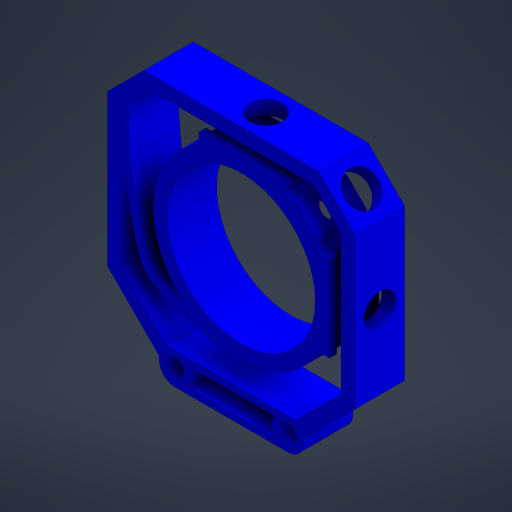
# Autodesk Inventor part: SM1 Lense Holder (V5)
Saved by Autodesk Inventor 2023.4 (Build 274418000, 418)
## iProperties
Created: 2022-07-25
Part Number: SM1 Lense Holder (V5)
Material: Generic
Document SubType Name: Modeling
Designer: xSibe
Density: 1 g/cm^3
Appearance: Plastic Blue
Author: xSibe
Autodesk Inventor part; units mm, degrees
ref_plane "YZ Plane" through (0, 0, 0) normal (1, 0, 0) x (0, 1, 0)
ref_plane "XZ Plane" through (0, 0, 0) normal (0, 1, 0) x (-1, 0, 0)
sketch "Sketch1" plane through (0, 0, 0) normal (0, 0, 1) x (1, 0, 0)
  circle A0 centre (139.6, 3.85) radius 2.8125
  circle A1 centre (159.6, 3.85) radius 2.8125
  line L0 (159.6, 1.0375) -> (139.6, 1.0375)
  line L1 (139.6, 2.145) -> (159.6, 2.145)
  line L2 (139.6, 5.555) -> (159.6, 5.555)
  line L3 (132.55, 24.9) -> (166.65, 24.9)
  line L4 (149.6, 24.9) -> (151.3678, 26.6678)
  line L5 (149.6, 24.9) -> (152.1, 24.9) construction
  circle A2 centre (151.3678, 26.6678) radius 13.125
  circle A3 centre (151.3678, 26.6678) radius 10.625
  circle A4 centre (151.3678, 26.6678) radius 15.625
  line L6 (151.3678, 26.6678) -> (151.3678, 42.2928)
  line L7 (151.3678, 42.2928) -> (151.3678, 41.2928)
  line L8 (143.8678, 40.2928) -> (158.8678, 40.2928)
  line L9 (158.8678, 40.2928) -> (158.8678, 42.2928)
  line L10 (158.8678, 42.2928) -> (143.8678, 42.2928)
  line L11 (143.8678, 42.2928) -> (143.8678, 40.2928)
  line L12 (143.8678, 40.2928) -> (158.8678, 42.2928) construction
  line L13 (158.8678, 40.2928) -> (143.8678, 42.2928) construction
  line L14 (151.3678, 26.6678) -> (162.4163, 37.7163)
  line L15 (162.4163, 37.7163) -> (161.9744, 37.2744)
  line L16 (164.8028, 36.5673) -> (161.2673, 40.1028)
  line L17 (161.2673, 40.1028) -> (159.1459, 37.9815)
  line L18 (159.1459, 37.9815) -> (162.6815, 34.4459)
  line L19 (162.6815, 34.4459) -> (164.8028, 36.5673)
  line L20 (164.8028, 36.5673) -> (159.1459, 37.9815) construction
  line L21 (161.2673, 40.1028) -> (162.6815, 34.4459) construction
  line L22 (164.8028, 36.5673) -> (169.8028, 36.5673) construction
  line L23 (164.9928, 19.1678) -> (164.9928, 34.1678)
  line L24 (164.9928, 34.1678) -> (166.9928, 34.1678)
  line L25 (166.9928, 34.1678) -> (166.9928, 19.1678)
  line L26 (166.9928, 19.1678) -> (164.9928, 19.1678)
  line L27 (151.3678, 42.2928) -> (151.3678, 44.2928)
  line L28 (166.9928, 26.6678) -> (168.9928, 26.6678)
  line L29 (139.3822, 5.4322) -> (159.8178, 5.4322)
  line L30 (169.0678, 14.6822) -> (169.0678, 39.3678)
  line L31 (164.0678, 44.3678) -> (135.1322, 44.3678)
  line L32 (130.1322, 39.3678) -> (130.1322, 14.6822)
  line L33 (130.1322, 5.4322) -> (169.0678, 44.3678) construction
  line L34 (169.0678, 5.4322) -> (130.1322, 44.3678) construction
  line L35 (139.3822, 5.4322) -> (130.1322, 14.6822)
  line L36 (159.8178, 5.4322) -> (169.0678, 14.6822)
  line L37 (164.0678, 44.3678) -> (169.0678, 39.3678)
  line L38 (135.1322, 44.3678) -> (130.1322, 39.3678)
  line L39 (134.0967, 46.8678) -> (127.6322, 40.4033)
  line L40 (127.6322, 40.4033) -> (127.6322, 13.6467)
  line L41 (127.6322, 13.6467) -> (138.3467, 2.9322)
  line L42 (138.3467, 2.9322) -> (160.8533, 2.9322)
  line L43 (160.8533, 2.9322) -> (171.5678, 13.6467)
  line L44 (171.5678, 13.6467) -> (171.5678, 40.4033)
  line L45 (171.5678, 40.4033) -> (165.1033, 46.8678)
  line L46 (165.1033, 46.8678) -> (134.0967, 46.8678)
  circle A5 centre (139.6, 3.85) radius 1.705
  circle A6 centre (159.6, 3.85) radius 1.705
  line L47 (151.3678, 11.0428) -> (133.8678, 11.0428)
  arc A7 (133.8678, 16.0428) -> (151.3678, 11.0428) centre (151.3678, 44.1678) ccw
  line L48 (133.8678, 11.0428) -> (133.8678, 16.0428)
  arc A8 (130.1322, 39.3678) -> (133.8678, 16.0428) centre (204.8217, 39.3678) ccw
  arc A9 (131.3931, 40.6286) -> (134.9138, 16.8679) centre (204.8217, 39.3678) ccw
  arc A10 (134.9138, 16.8679) -> (143.1729, 13.3642) centre (151.3678, 44.1678) ccw
  arc A11 (133.1269, 18.4305) -> (136.1735, 14.7331) centre (138.9617, 20.1344) ccw
  line L49 (133.8678, 16.0428) -> (133.1269, 18.4305)
  line L50 (134.9138, 16.8679) -> (134.1885, 19.2604)
  arc A12 (134.1885, 19.2604) -> (137.2433, 15.593) centre (139.8532, 20.8729) ccw
  line L51 (132.55, 7.7) -> (132.55, 42.1) projected
  line L52 (166.65, 7.7) -> (166.65, 42.1) projected
  circle A13 centre (139.6, 3.85) radius 1.5625 projected
  circle A14 centre (159.6, 3.85) radius 1.5625 projected
  line L53 (138.152, 6.6625) -> (161.048, 6.6625)
  point P0 (0, 0)
  point P1 (56.6078, -34.1566)
  point P2 (141.8368, 2.145)
  point P3 (141.8368, 5.555)
  point P4 (157.3632, 5.555)
  point P5 (157.3632, 2.145)
  point P6 (156.9415, 2.9322)
  point P7 (142.2585, 2.9322)
  point P8 (138.4142, 6.4003)
  point P9 (160.7858, 6.4003)
  point P10 (143.8678, 40.3751)
  point P11 (165.0751, 19.1678)
  point P12 (165.0751, 34.1678)
  point P13 (164.0417, 35.8062)
  point P14 (160.5062, 39.3417)
  point P15 (158.8678, 40.3751)
  point P16 (162.3519, 4.4308)
  point P17 (136.8481, 4.4308)
  point P18 (-7.8312, 14.244)
  point P19 (157.2748, 5.4322)
  point P20 (141.9252, 5.4322)
  point P21 (133.1872, 18.2361)
  point P22 (134.2467, 19.0685)
  point P23 (132.8214, 24.9)
  point P24 (166.9928, 26.6678)
  point P25 (166.65, 41.7855)
  point P26 (166.65, 34.1678)
  point P27 (166.65, 19.1678)
  point P28 (166.65, 12.2645)
  dimension "d2" = 2.5
  dimension "d3" = 45
  dimension "d4" = 26.25
  dimension "d5" = 2.5
  dimension "d6" = 2.5
  dimension "d7" = 1
  dimension "d8" = 15
  dimension "d9" = 2
  dimension "d10" = 0.625
  dimension "d11" = 5
  dimension "d12" = 135
  dimension "d13" = 3
  dimension "d14" = 2
  dimension "d15" = 2
  dimension "d16" = 38.9355
  dimension "d17" = 38.9355
  dimension "d18" = 9.25
  dimension "d19" = 9.25
  dimension "d20" = 9.25
  dimension "d21" = 9.25
  dimension "d22" = 5
  dimension "d23" = 5
  dimension "d24" = 5
  dimension "d25" = 5
  dimension "d26" = 2.5
  dimension "d48" = 17.5
  dimension "d49" = 5
  dimension "d50" = 1.25
  dimension "d51" = 2.5
  dimension "d52" = 2.5
  dimension "d56" = 0.1425
  dimension "d57" = 0.1425
  dimension "d58" = 1.25
  dimension "d59" = 1.25
  constraints: 104 end point, 24 point on circle, 15 point on line, 11 centre point, 11 tangent, 10 horizontal, 10 midpoint, 8 parallel, 6 perpendicular, 4 symmetric about line, 3 coincident, 2 equal length, 2 vertical, 14 other
  measures "d2" distance of L4.start L4.end
  measures "d3" angle of L5 L4
  measures "d4" diameter of A2
  measures "d5" radial gap between concentric circles of A2 A3
  measures "d6" radial gap between concentric circles of A2 A4
  measures "d7" distance of L6.end L7.end
  measures "d8" distance of L10.end L9.end
  measures "d9" distance of L9.end L8.end
  measures "d10" distance of L14.end L15.end
  measures "d11" distance of L16.start L16.end
  measures "d12" angle of L22 L16
  measures "d13" distance of L17.end L16.end
  measures "d14" distance of L6.end L27.end
  measures "d15" distance of L28.start L28.end
  measures "d16" distance of L33.end L34.end
  measures "d17" distance of L34.end L33.start
  measures "d18" distance of L29.start L33.start
  measures "d19" distance of L32.end L33.start
  measures "d20" distance of L29.end L34.start
  measures "d21" distance of L30.start L34.start
  measures "d22" distance of L31.start L33.end
  measures "d23" distance of L30.end L33.end
  measures "d24" distance of L31.end L34.end
  measures "d25" distance of L32.start L34.end
  measures "d26" distance between parallel lines of L31 L46
  measures "d48" distance of L47.start L47.end
  measures "d49" distance of L47.end L48.end
  measures "d50" radial gap between concentric circles of A8 A9
  measures "d51" distance of L48.end L49.end
  measures "d52" distance of L50.start L50.end
  measures "d56" radial gap between concentric circles of A6 A14
  measures "d57" radial gap between concentric circles of A5 A13
extrude "Extrusion1" add sketch "Sketch1" along normal mid plane 8.75 contours A0 L42 A5 L29 | L29 A5 L2 A0 | A0 L2 A1 L29 | A0 L1 A5 L42 | L2 A5 L35 A0 | A0 L53 A1 L2 | L29 A6 L42 A1 | A1 L2 A6 L29 | L1 A1 L0 A0 | A0 L41 A5 L1 | L42 A6 L1 A1 | A0 L35 L53 | A1 L36 A6 L2 | L1 A6 L43 A1 | L35 A5 L41 A0 | A0 L41 L51 L35 | L53 L36 A1 | L51 L41 L40 L39 L46 L45 L44 L43 L52 L36 L30 L37 L31 L38 L32 L35 | L36 L52 L43 A1 | A1 L43 A6 L36 | L51 L3 A9 A10 A4 A7 A11 A8 | A8 L38 A9 L51 | L51 A9 L3 | L52 A4 L25 L26 | L26 A4 L52 | A12 A10 L50 | L26 L23 L3 L52 A4 | A4 L3 A2 L23 L26 | L52 A4 | A4 L11 L8 L6 A2 L3 | L50 A9 | A4 L52 L24 L25 | L3 L23 L24 A4 L52 | L11 L10 A4 | A4 L6 L8 L11 | L52 A4 L24 | L3 A2 L14 L18 L19 A4 L24 L23 | L6 L8 L9 A4 L17 L18 L14 A2 | L10 L9 A4 | A4 L9 L8 L6 | L19 L18 L14 A4 | A4 L17 L16 L19 | L18 L17 A4 L14
sketch "Sketch2" plane through (0, 0, 0) normal (0, 0, 1) x (1, 0, 0)
  circle A0 centre (151.3678, 26.6678) radius 13.125 projected
  circle A1 centre (151.3678, 26.6678) radius 11.25
  point P0 (0, 0)
  dimension "d30" = 1.875
  constraints: 1 centre point
  measures "d30" radial gap between concentric circles of A0 A1
extrude "Extrusion2" [suppressed]
sketch "Sketch3" plane through (171.5678, 13.6467, -4.375) normal (1, 0, 0) x (0, 0, -1)
  line L0 (0, 5.5211) -> (-8.75, 5.5211) projected
  line L1 (0, 20.5211) -> (0, 5.5211) projected
  line L2 (0, 20.5211) -> (-8.75, 20.5211) projected
  line L3 (-8.75, 5.5211) -> (-8.75, 20.5211) projected
  line L4 (-4.375, 20.5211) -> (-4.375, 5.5211)
  circle A0 centre (-4.375, 13.0211) radius 2.875
  point P0 (-4.375, -13.6467)
  dimension "d33" = 5.75
  constraints: 3 midpoint, 2 end point, 1 centre point
  measures "d33" diameter of A0
extrude "Extrusion3" cut sketch "Sketch3" against normal up to surface (2.5 mm away) contours A0 L4 | L4 A0
sketch "Sketch4" plane through (165.0751, 34.1678, -4.375) normal (0, 1, 0) x (1, 0, 0)
  line L0 (0, 0) -> (1.9177, 0) projected
  line L1 (0, 0) -> (0, -8.75) projected
  line L2 (1.9177, -8.75) -> (0, -8.75) projected
  line L3 (1.9177, -8.75) -> (0, -8.75)
  line L4 (0, -8.75) -> (0, -7.5)
  line L5 (0, -7.5) -> (1.9177, -7.5)
  line L6 (1.9177, -7.5) -> (1.9177, -8.75)
  line L7 (1.9177, -7.5) -> (0, -5.5823)
  line L8 (1.9177, -7.5) -> (4.6297, -7.5) construction
  line L9 (0, -4.375) -> (1.9177, -4.375)
  line L10 (1.9177, -1.25) -> (0, -3.1677)
  line L11 (0.9588, -8.75) -> (0.9588, 0)
  line L12 (1.9177, 0) -> (1.9177, -8.75) projected
  point P0 (-165.0751, -4.375)
  point P1 (0.9588, -2.2088)
  point P2 (0.9588, -6.5412)
  dimension "d36" = 1.25
  dimension "d37" = 135
  constraints: 18 end point, 4 point on line, 3 midpoint, 2 horizontal, 2 parallel, 2 symmetric about line, 1 equal length, 1 perpendicular
  measures "d36" distance of L3.end L4.end
  measures "d37" angle of L8 L7
extrude "Extrusion4" cut sketch "Sketch4" against normal up to surface (15 mm away) contours L10 L12 L9 L11 | L9 L12 L7 L11
ref_plane "Work Plane1" through (166.9928, 42.2928, 4.375) normal (0.7071068, -0.7071068, 0) x (0, 0, -1)
mirror "Mirror1" about plane through (166.9928, 42.2928, 4.375) normal (0.7071068, -0.7071068, 0) of "Extrusion3", "Extrusion4"
sketch "Sketch5" plane through (171.5678, 40.4033, 4.375) normal (0.7071068, 0.7071068, 0) x (0.7071068, -0.7071068, 0)
  line L0 (0, 8.75) -> (0, 0) projected
  line L1 (-9.1421, 8.75) -> (0, 8.75) projected
  line L2 (-9.1421, 8.75) -> (-9.1421, 0) projected
  line L3 (0, 0) -> (-9.1421, 0) projected
  line L4 (-2.0711, 8.75) -> (-2.0711, 0) projected
  line L5 (-7.0711, 8.75) -> (-2.0711, 8.75) projected
  line L6 (-7.0711, 8.75) -> (-7.0711, 0) projected
  line L7 (-2.0711, 0) -> (-7.0711, 0) projected
  circle A0 centre (-4.5711, 4.375) radius 1.875
  line L8 (-7.0711, 4.375) -> (-2.0711, 4.375)
  circle A1 centre (-4.5711, 4.375) radius 3
  point P0 (-92.7473, 4.375)
  dimension "d40" = 3.75
  dimension "d41" = 6
  constraints: 3 midpoint, 2 centre point, 2 end point, 1 coincident
  measures "d40" diameter of A0
  measures "d41" diameter of A1
extrude "Extrusion5" cut sketch "Sketch5" against normal up to surface (2.5 mm away) contours A1 L4 | L4 L8 A0 L6 A1 | A1 L6 L8 A0 L4 | L6 A1 | L8 A0 | A0 L8
extrude "Extrusion6" cut sketch "Sketch5" against normal up to next from surface at -7.496 contours L8 A0 | A0 L8
chamfer "Chamfer1" distance 1.075 angle 45 2 edges at (164.0417, 35.8062, 0) (160.5062, 39.3417, 0)
equation "\"d19\" = d18"
equation "\"d20\" = d18"
equation "\"d21\" = d20"
equation "\"d23\" = d22"
equation "\"d24\" = d22"
equation "\"d25\" = d24"
body "Solid1"
